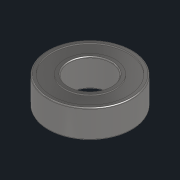
# Autodesk Inventor part: MR126ZZ
Saved by Autodesk Inventor 2022 (Build 260153000, 153)
## iProperties
Category: PARTsolutions
Company: MISUMI
Part Number: MR126ZZ
Material: 鋼、炭素鋼
Catalog Web Link: www.cadenas.de
Description: ミスミ
Vendor: MISUMI
Document SubType Name: Modeling
Designer: partserver
Manufacturer: MISUMI
Mass: 2.494 g
Surface Area: 4.11305 cm^2
Volume: 0.317707 cm^3
Density: 7.85 g/cm^3
Appearance: 半つや出し
PSOL_IDENT_0: {$CADENAS_DATA\23d-libs\misumi\metric\12_bearing_holders\sutb692zz.prj},169 {VTYP=3D},{NB=SUTB126A4Z
PSOL_IDENT_1: Z},{LINA=SUTB126A4ZZ},{NN=SUTB_ _ _ ZZ},{DATE=09.09.2019 09:02:54},{GEOMDATE=25.05.2017 07:46:04},{V
PSOL_IDENT_2: ERSION=},{LINEID=160},{WBVAR=},{WBNUMERIC=}  {NB=SUTB126A4ZZ},{LINA=SUTB126A4ZZ},{KT=DUMMY},{PN=SUTB
PSOL_IDENT_3: 126A4ZZ},{TYPE=SUTB126A4ZZ},{BN=126A4ZZ},{DD=6},{D=12},{B=4.0},{RR=0.15},{B11=0.20},{D11=7.20},{D22=
PSOL_IDENT_4: 10.90},{CR=610},{COR=234},{RRPPMM=43000},{DS=7.2},{DDHH=10.9},{R=0.15},{MASS=1.74}
NB: SUTB126A4ZZ
NN: SUTB_ _ _ ZZ
NT: Prustro  Miniature Ball Bearings -Double Shield Type-
NBSYN: $PN.
LINA: SUTB126A4ZZ
CATALOG: Misumi
PN: SUTB126A4ZZ
BN: 126A4ZZ
DD: 6
D: 12
B: 4
RR: 0.15
CR: 610
COR: 234
RRPPMM: 43000
DS: 7.2
DDHH: 10.9
R: 0.15
MASS: 1.74
SUPPLIER: MISUMI
ARTICLENO: SUTB126A4ZZ
BOMINFO: SUTB126A4ZZ
CREATOR: CADENAS GmbH
Title: SUTB126A4ZZ
Author: Cadenas PARTsolutions
Comments: Prustro  Miniature Ball Bearings -Double Shield Type-
Autodesk Inventor part; units mm, degrees
sketch "Sketch_1" plane through (0, 0, 0) normal (1, 0, 0) x (0, 0, -1)
  line L0 (4, 0) -> (0, 0)
  arc A0 (0, 3.15) -> (0.15, 3) centre (0.15, 3.15) ccw
  line L1 (0.15, 3) -> (3.85, 3)
  arc A1 (3.85, 3) -> (4, 3.15) centre (3.85, 3.15) ccw
  line L2 (4, 3.15) -> (4, 3.6)
  line L3 (4, 3.6) -> (3.8, 3.6)
  line L4 (3.8, 3.6) -> (3.8, 5.45)
  line L5 (3.8, 5.45) -> (4, 5.45)
  line L6 (4, 5.45) -> (4, 5.85)
  arc A2 (4, 5.85) -> (3.85, 6) centre (3.85, 5.85) ccw
  line L7 (3.85, 6) -> (0.15, 6)
  arc A3 (0.15, 6) -> (0, 5.85) centre (0.15, 5.85) ccw
  line L8 (0, 5.85) -> (0, 5.45)
  line L9 (0, 5.45) -> (0.2, 5.45)
  line L10 (0.2, 5.45) -> (0.2, 3.6)
  line L11 (0.2, 3.6) -> (0, 3.6)
  line L12 (0, 3.6) -> (0, 3.15)
  constraints: 26 end point, 8 point on circle, 4 centre point
revolve "Revolution1" add sketch "Sketch_1" angle 360 about axis through (0, 0, -4) along (0, 0, -1)
ref_plane "to_housing_XY" through (0, 0, 0) normal (0, 0, -1) x (1, 0, 0)
ref_plane "to_housing_YZ" through (0, 0, 0) normal (1, 0, 0) x (0, -1, 0)
ref_plane "to_housing_ZX" through (0, 0, 0) normal (0, -1, 0) x (0, 0, -1)
body "Solid1"
